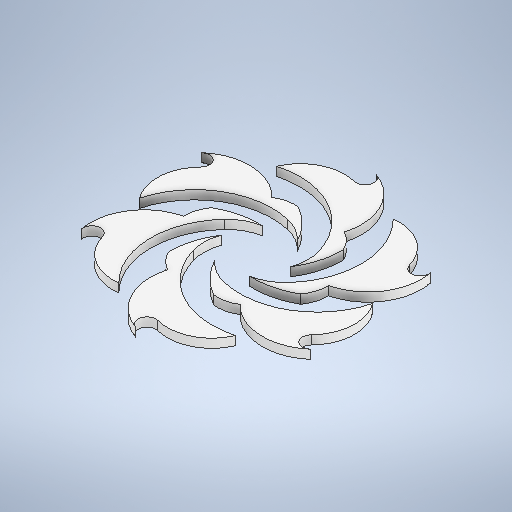
# Autodesk Inventor part: LOGO
Saved by Autodesk Inventor 2026.1 (Build 301233020, 233B)
## iProperties
Created: 2025-07-18
Part Number: LOGO
Material: 一般
Document SubType Name: Modeling
Designer: hibik
Density: 1 g/cm^3
Appearance: 既定
Author: hibik
Autodesk Inventor part; units mm, degrees
ref_plane "YZ Plane" through (0, 0, 0) normal (1, 0, 0) x (0, 1, 0)
ref_plane "XZ Plane" through (0, 0, 0) normal (0, 1, 0) x (-1, 0, 0)
sketch "スケッチ1" plane through (0, 0, 0) normal (0, 1, 0) x (-1, 0, 0)
  circle A0 centre (0, 0) radius 37.5 construction
  arc A1 (-9.4224, 1.9643) -> (7.3361, -6.2308) centre (0, 0) ccw
  arc A2 (-9.4224, 1.9643) -> (21.7871, -22.0595) centre (11.9922, -2.5) ccw
  arc A3 (7.3361, -6.2308) -> (21.7871, -22.0595) centre (6.6708, -21.3491) ccw
  arc A4 (3.125, -30.8531) -> (1.6746, -35.6335) centre (2.5, -33.2737) ccw
  arc A5 (7.283, -6.2928) -> (17.7717, -23.5977) centre (6.25, -18.75) ccw
  arc A6 (-12.0923, -12.5) -> (-9.8739, -1.8751) centre (-3.5, -8.75) ccw
  arc A7 (-8.75, -1) -> (-8.9465, -8.8314) centre (3.0185, -5.2135) ccw
  arc A8 (-8.75, -1) -> (-12.0923, -12.5) centre (9.1576, -12.4403) ccw
  point P0 (-7.8413, -17.0592)
  point P1 (6.6984, -142.534)
  point P2 (12.5, -123.4123)
  point P3 (71.0869, -94.3908)
  point P4 (-3.3189, -18.1233)
  point P5 (-6.2079, -17.7254)
  point P6 (-5.7595, -15.2826)
  point P7 (-39.4956, -7.5004)
  point P8 (87.1485, -88.2381)
  point P9 (5.5379, -6.2586)
  point P10 (-6.5853, -14.0496)
  point P11 (4.252, -6.4107)
  point P12 (5.5411, -6.2701)
  point P13 (-9.5, -1.5464)
  point P14 (-2.0507, -9.404)
  point P15 (63.4693, -48.0608)
  point P16 (-9.2313, -2.7247)
  point P17 (-9.397, -2.0823)
  point P18 (-9.8772, -2.9937)
  point P19 (-36.7334, -7.086)
  point P20 (-37.6897, 7.8571)
  point P21 (-35.7696, -6.328)
  point P22 (5.8128, -7.6715)
  point P23 (-2.4835, -9.2991)
  dimension "d0" = 75
  dimension "d1" = 19.25
  dimension "d7" = 5
  dimension "d9" = 6.25
  dimension "d10" = 18.75
  dimension "d11" = 25
  dimension "d13" = 18.75
  dimension "d15" = 8.75
  dimension "d16" = 3.5
  dimension "d17" = 2.5
  dimension "d18" = 2.5
  dimension "d19" = 43.75
  dimension "d20" = 8.75
  dimension "d21" = 1
  dimension "d23" = 3.75
  dimension "d24" = 21.25
  dimension "d25" = 12.5
  constraints: 22 point on circle, 9 centre point, 6 tangent, 2 coincident
  measures "d0" diameter of A0
  measures "d1" diameter of A1
  measures "d7" diameter of A4
  measures "d9" horizontal distance of point (0, 0) A5.centre
  measures "d10" vertical distance of point (0, 0) A5.centre
  measures "d11" diameter of A5
  measures "d13" diameter of A6
  measures "d15" vertical distance of point (0, 0) A6.centre
  measures "d16" horizontal distance of point (0, 0) A6.centre
  measures "d17" vertical distance of point (0, 0) A2.centre
  measures "d18" horizontal distance of point (0, 0) A4.centre
  measures "d19" diameter of A2
  measures "d20" horizontal distance of point (0, 0) A7.start
  measures "d21" vertical distance of A7.start point (0, 0)
  measures "d23" vertical distance of A6.centre A6.start
  measures "d24" radius of A8
  measures "d25" radius of A7
extrude "押し出し1" add sketch "スケッチ1" along normal blind 2.5 contours A6 A5 A2 | A2 A5 A6 | A5 A6 A3 A2 | A5 A4 A3 A6 | A8 A7 A1 | A1 A7 A2 A8 | A3 A6 A8 A2
pattern_circular "円形状パターン1" count 6 over 360 about axis through (0, -10, 0) along (0, 1, 0) of "押し出し1"
sketch "スケッチ2" plane through (3.831, 2.5, 11.6355) normal (0, 1, 0) x (0.9998, 0, -0.0187)
  line L0 (-9.232, 3.8908) -> (-13.1897, 12.6644)
  line L1 (-13.1897, 12.6644) -> (-7.5705, 20.4788)
  line L2 (-7.5705, 20.4788) -> (2.0066, 19.5195)
  line L3 (2.0066, 19.5195) -> (5.9644, 10.7459)
  line L4 (5.9644, 10.7459) -> (0.3451, 2.9315)
  line L5 (0.3451, 2.9315) -> (-9.232, 3.8908)
  circle A0 centre (-3.6127, 11.7052) radius 9.625
  point P0 (-7.2722, 3.6945)
  point P1 (-12.3798, 10.8691)
  point P2 (-8.7204, 18.8797)
  point P3 (0.0468, 19.7158)
  point P4 (5.1545, 12.5413)
  point P5 (1.495, 4.5306)
  dimension "d27" = 19.25
  constraints: 12 end point, 2 coincident, 1 point on line, 16 other
ref_plane "作業平面1" through (4.1212, 2.5, 8.698) normal (0.081, 0, -0.9967) x (-0.9967, 0, -0.081)
equation "\"r\" = 75"
